54644ffa-fdaa-45b0-811d-ef362eb34d84 (Autodesk Fusion 360 design; units mm, degrees)
Autodesk Fusion 360 part; units mm, degrees
sketch "Sketch2" plane through (0, 0, 0) normal (1, 0, 0) x (0, 1, 0)
  line L0 (0, 0) -> (23.0124, 0) construction
  line L1 (46.6852, 0) -> (23.0124, 0) construction
  circle A0 centre (34.8488, 0) radius 11.8364
  dimension "d1" = 23.0124
  dimension "d2" = 46.6852
  constraint coincident L0.start origin
  constraint horizontal L0
  constraint parallel L0 L1
  constraint midpoint L1 A0.centre
  constraint coincident L1.start A0
  measures "d1" distance of L0.start L0.end
  measures "d2" distance of L0.start L1.start
revolve "Revolve4" add sketch "Sketch2" angle 360 about axis through (0, 0, 1.75) along (0, 0, 1) makes body 1
ref_plane "WorkPlane1" through (-46.6852, 0, 0) normal (1, 0, 0) x (0, 1, 0)
ref_plane "WorkPlane2" through (96.1898, 0, 0) normal (1, 0, 0) x (0, 1, 0)
ref_plane "WorkPlane3" through (32.6898, 0, 0) normal (1, 0, 0) x (0, 1, 0)
sketch "Sketch6" plane through (32.6898, 0, 0) normal (1, 0, 0) x (0, 1, 0)
  circle A0 centre (0, 0) radius 12.7
  dimension "d31" = 25.4
  constraint coincident A0.centre origin
  measures "d31" diameter of A0
extrude "Extrude1" add sketch "Sketch6" along normal up to surface (63.5 mm away) separate body makes body 2
ref_plane "WorkPlane4" through (34.8488, 0, 0) normal (1, 0, 0) x (0, 1, 0)
sketch "Sketch7" plane through (0, 0, 0) normal (0, 0, 1) x (1, 0, 0)
  line L0 (34.8488, 0.75) -> (34.8488, 21.75)
  line L1 (0, 0) -> (76.2, 0) construction
  line L2 (34.8488, 18.7283) -> (34.8488, -25.4) construction
  line L3 (34.8488, 0) -> (72.9488, 0)
  line L4 (72.9488, 0) -> (72.9488, 22.5034)
  line L5 (34.8488, 0) -> (34.8488, 12.7)
  line L6 (65.7205, 27.1068) -> (34.8488, 12.7)
  arc A0 (72.9488, 22.5034) -> (65.7205, 27.1068) centre (67.8688, 22.5034) ccw
  point P0 (72.9488, 30.48)
  dimension "d40" = 38.1
  dimension "d41" = 30.48
  dimension "d42" = 12.7
  dimension "d43" = 5.08
  constraint coincident L1.start origin
  constraint horizontal L1
  constraint coincident L0 L2.start
  constraint parallel L0 L2
  constraint coincident L2 L3.start
  constraint coincident L1 L3.start
  constraint perpendicular L2 L3
  constraint perpendicular L3 L4
  constraint perpendicular L3 L5
  constraint coincident P0 L4
  constraint coincident P0 L6
  constraint tangent L4 A0
  constraint tangent L6 A0
  measures "d40" distance of L3.start L3.end
  measures "d41" distance of L3.end P0
  measures "d42" distance of L3.start L5.end
  measures "d43" radius of A0
revolve "Revolve5" add sketch "Sketch7" angle 360 about axis through (0, 0, 0) along (1, 0, 0) bodies 1 2
thread "Thread2" "ANSI Unified Screw Threads 0.3125 5/16-18 UNC 3A" major diameter 7.8283 minor diameter 6.2586 pitch 1.4111 angle 60 modelled right hand crest width 0.2172 on face at (80.6958, 12.5355, 2.0372) crest through (72.596, 3.9141, 0) on bodies 1
fillet "Fillet2" radius 5.08 2 edges at (43.5654, -16.7635, -0.3753) (43.5654, 16.7635, 0.3753) on bodies 1
equation "d27 = -d2"
equation "d28 = 5.625 in"
equation "d30 = -2.500 in"
equation "EyeInner = d1"
equation "EyeOuter = d2"
equation "ThreadDia = d31"
equation "TotalLength = d28"
equation "ShankLength = d30"
equation "d39 = d1 + ( ( d2 - d1 ) ) / 2"
equation "d40 = d31 * 1.5"
equation "d41 = d31 * 1.2"
equation "d42 = d31 / 2"
equation "d43 = d31 * 0.2"
equation "d45 = d31 * 0.2"
